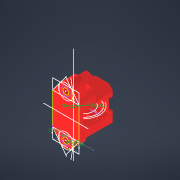
# Autodesk Inventor part: Front-Idlers_Inlet
Saved by Autodesk Inventor 2022.1 (Build 261234000, 234)
## iProperties
Created: 2021-09-01
Part Number: Front-Idlers_Inlet
Material: Generisch
Document SubType Name: Modeling
Designer: Rama
Density: 1 g/cm^3
Appearance: Hellrot
Author: Rama
Autodesk Inventor part; units mm, degrees
ref_plane "YZ Plane" through (0, 0, 0) normal (1, 0, 0) x (0, 1, 0)
ref_plane "XZ Plane" through (0, 0, 0) normal (0, 1, 0) x (-1, 0, 0)
ref_plane "XY Plane" through (0, 0, 0) normal (0, 0, 1) x (1, 0, 0)
sketch "Skizze1" plane through (0, 0, 0) normal (0, 0, 1) x (1, 0, 0)
  line L0 (-7.5, 9) -> (7.5, 9)
  line L1 (7.5, 9) -> (7.5, -9)
  line L2 (7.5, -9) -> (-7.5, -9)
  line L3 (-7.5, -9) -> (-7.5, 9)
  line L4 (-7.5, 9) -> (7.5, -9) construction
  line L5 (7.5, 9) -> (-7.5, -9) construction
  point P0 (0, 0)
  dimension "d0" = 15
  dimension "d1" = 18
  constraints: 12 end point, 2 midpoint, 2 parallel, 1 horizontal, 1 perpendicular
  measures "d0" distance of L1.end L2.end
  measures "d1" distance of L0.end L1.end
extrude "Extrusion1" add sketch "Skizze1" along normal blind 24
sketch "Skizze2" plane through (-7.5, 9, 0) normal (0, 1, 0) x (1, 0, 0)
  line L0 (0, -24) -> (15, -24) projected
  circle A0 centre (7.5, -14) radius 2.5
  point P0 (7.5, 0)
  dimension "d5" = 5
  dimension "d13" = 10
  constraints: 1 centre point
  measures "d5" diameter of A0
  measures "d13" distance from line of L0 A0.centre
extrude "Extrusion2" cut sketch "Skizze2" against normal through all
ref_plane "Arbeitsebene1" through (-7.5, 0, 0) normal (0, 1, 0) x (1, 0, 0)
sketch "Skizze3" plane through (-7.5, 0, 0) normal (0, 1, 0) x (1, 0, 0)
  circle A0 centre (7.5, -14) radius 2.5 projected
  circle A1 centre (7.5, -14) radius 8
  circle A2 centre (7.5, -14) radius 9
  line L0 (-1.5, -14) -> (16.5, -14)
  circle A3 centre (7.5, -14) radius 5
  line L1 (12.5, -14) -> (12.5, 0)
  line L2 (0, 0) -> (15, 0) projected
  line L3 (2.5, -14) -> (2.5, 0)
  line L4 (16.5, -14) -> (16.5, 0)
  line L5 (16.5, 0) -> (12.5, 0)
  line L6 (-1.5, -14) -> (-1.5, 0)
  line L7 (-1.5, 0) -> (2.5, 0)
  point P0 (7.5, 0)
  point P1 (15, 0)
  point P2 (12.5, -7.755)
  point P3 (2.5, -7.755)
  point P4 (0, 0)
  dimension "d8" = 16
  dimension "d9" = 18
  dimension "d10" = 10
  constraints: 14 end point, 5 point on line, 4 point on circle, 3 centre point, 3 coincident, 3 tangent, 2 parallel, 2 perpendicular, 1 collinear, 1 horizontal, 1 vertical
  measures "d8" diameter of A1
  measures "d9" diameter of A2
  measures "d10" diameter of A3
extrude "Extrusion3" cut sketch "Skizze3" against normal mid plane 10 contours L0 A3 A0 | A0 L0 A3 | L1 A1 L0 | L0 A1 A3 | A3 L3 A1 L1 | L0 A1 L3 | L0 A2 A1 | A1 L1 A2 L0 | L0 A2 L3 A1 | A2 L1 L2 L5 L4 | L6 L7 L2 L3 A2
sketch "Skizze4" plane through (-7.5, 9, 0) normal (0, 1, 0) x (1, 0, 0)
  line L0 (15, 0) -> (0, 0)
  line L1 (0, 0) -> (0, -4.5)
  line L2 (0, -4.5) -> (15, -4.5)
  line L3 (15, -4.5) -> (15, 0)
  circle A0 centre (7.5, -14) radius 2.5 projected
  line L4 (15, 0) -> (0, 0) projected
  line L5 (0, 0) -> (0, -24) projected
  line L6 (15, -24) -> (0, -24) projected
  line L7 (15, 0) -> (15, -24) projected
  line L8 (0, 0) -> (0, -24) projected
  line L9 (15, 0) -> (15, -24) projected
  line L10 (15, 0) -> (0, 0) projected
  line L11 (0, -18.9749) -> (0, 0) projected
  arc A1 (0, -18.9749) -> (15, -18.9749) centre (7.5, -14) ccw projected
  line L12 (15, 0) -> (15, -18.9749) projected
  line L13 (12.5, 0) -> (15, 0) projected
  line L14 (12.5, -7.755) -> (12.5, 0) projected
  arc A2 (12.5, -7.755) -> (2.5, -7.755) centre (7.5, -14) ccw projected
  line L15 (2.5, 0) -> (2.5, -7.755) projected
  line L16 (0, 0) -> (2.5, 0) projected
  circle A3 centre (7.5, -14) radius 2.5 projected
  point P0 (7.5, 0)
  point P1 (0, -2.25)
  point P2 (15, -2.25)
  point P3 (7.5, 0)
  dimension "d14" = 1.5
  constraints: 8 end point, 4 midpoint, 2 parallel, 2 point on line, 1 horizontal, 1 perpendicular
  measures "d14" distance edge to line of A2 L2
extrude "Extrusion4" cut sketch "Skizze4" against normal through all contours L3 L2 L14 L0 | L14 L2 L15 L0 | L15 L2 L1 L0
sketch "Skizze5" plane through (0, 0, 24) normal (0, 0, 1) x (1, 0, 0)
  line L0 (-3.5, 15) -> (3.5, 15)
  line L1 (3.5, 15) -> (3.5, -15)
  line L2 (3.5, -15) -> (-3.5, -15)
  line L3 (-3.5, -15) -> (-3.5, 15)
  line L4 (-3.5, 15) -> (3.5, -15) construction
  line L5 (3.5, 15) -> (-3.5, -15) construction
  line L6 (-7.5, -9) -> (7.5, -9) projected
  line L7 (7.5, -9) -> (7.5, 9) projected
  line L8 (7.5, 9) -> (-7.5, 9) projected
  line L9 (-7.5, 9) -> (-7.5, -9) projected
  point P0 (0, 0)
  point P1 (3.5, -9)
  point P2 (-3.5, -9)
  point P3 (-3.5, 9)
  point P4 (3.5, 9)
  dimension "d17" = 7
  dimension "d18" = 30
  constraints: 12 end point, 2 midpoint, 2 parallel, 1 horizontal, 1 perpendicular
  measures "d17" distance of L1.end L2.end
  measures "d18" distance of L0.end L1.end
extrude "Extrusion5" add sketch "Skizze5" against normal blind 7.5 contours L0 L1 L8 L3 | L6 L1 L2 L3
sketch "Skizze6" plane through (0, 0, 16.5) normal (0, 0, -1) x (-1, 0, 0)
  line L0 (3.5, 9) -> (3.5, 15) projected
  line L1 (3.5, 15) -> (-3.5, 15) projected
  line L2 (-3.5, 15) -> (-3.5, 9) projected
  line L3 (0, 9) -> (-3.5, 9) projected
  line L4 (3.5, 9) -> (0, 9) projected
  line L5 (-3.5, -9) -> (-3.5, -15) projected
  line L6 (-3.5, -15) -> (3.5, -15) projected
  line L7 (3.5, -15) -> (3.5, -9) projected
  line L8 (0, -9) -> (3.5, -9) projected
  line L9 (-3.5, -9) -> (0, -9) projected
  line L10 (3.5, 9) -> (3.5, 15) projected
  line L11 (-3.5, 9) -> (3.5, 9)
  line L12 (3.5, 9) -> (3.5, 15)
  line L13 (3.5, 15) -> (-3.5, 15)
  line L14 (-3.5, 15) -> (-3.5, 9)
  line L15 (-3.5, 9) -> (3.5, 15) construction
  line L16 (3.5, 9) -> (-3.5, 15) construction
  line L17 (-3.5, -15) -> (3.5, -15) projected
  line L18 (-3.5, -9) -> (3.5, -9)
  line L19 (3.5, -9) -> (3.5, -15)
  line L20 (3.5, -15) -> (-3.5, -15)
  line L21 (-3.5, -15) -> (-3.5, -9)
  line L22 (-3.5, -9) -> (3.5, -15) construction
  line L23 (3.5, -9) -> (-3.5, -15) construction
  point P0 (0, 0)
  point P1 (0, 12)
  point P2 (0, -12)
  constraints: 24 end point, 4 midpoint, 4 parallel, 2 horizontal, 2 perpendicular
hole "Bohrung1" at (0, 12, 16.5) at (0, -12, 16.5) direction (0, 0, 1) diameter 3.3 end through all counterbore diameter 4.8 counterbore depth 3.8
sketch "Skizze7" plane through (-7.5, 9, 4.5) normal (0, 1, 0) x (1, 0, 0)
  line L0 (5.6485, 8.9497) -> (5.6485, -0.1503)
  spline S0 degree 3 poles (5.6485, -0.1503) (5.6485, -0.2757) (5.6235, -0.4093) (5.5221, -0.6548) (5.4458, -0.7666) (5.2684, -0.9452) (5.1549, -1.0229) (4.9074, -1.1255) (4.7734, -1.1503) (4.6485, -1.1503) knots 0 0 0 0 0.247012 0.247012 0.494023 0.494023 0.747012 0.747012 1 1 1 1
  line L1 (2.6485, -1.1503) -> (4.6485, -1.1503)
  spline S1 degree 3 poles (2.4137, -1.1224) (2.359, -1.1092) (2.3053, -1.0913) (2.1283, -1.0152) (2.0153, -0.935) (1.845, -0.7571) (1.7725, -0.6496) (1.6741, -0.4099) (1.6485, -0.2772) (1.6485, -0.1503) knots 0 0 0 0 0.128043 0.128043 0.438246 0.438246 0.719123 0.719123 1 1 1 1
  spline S2 degree 3 poles (2.6485, -1.1503) (2.5718, -1.1503) (2.4922, -1.1413) (2.4137, -1.1224) knots 0 0 0 0 1 1 1 1
  line L2 (1.6485, -0.1503) -> (1.6485, 8.9497)
  spline S3 degree 3 poles (1.6485, 8.9497) (1.6485, 9.0766) (1.6741, 9.2092) (1.7725, 9.449) (1.845, 9.5564) (2.0153, 9.7344) (2.1283, 9.8145) (2.3053, 9.8906) (2.359, 9.9085) (2.4137, 9.9217) knots 0 0 0 0 0.280877 0.280877 0.561754 0.561754 0.871957 0.871957 1 1 1 1
  line L3 (4.6485, 9.9497) -> (2.6485, 9.9497)
  spline S4 degree 3 poles (4.6485, 9.9497) (4.7734, 9.9497) (4.9074, 9.9248) (5.1549, 9.8223) (5.2684, 9.7446) (5.4458, 9.566) (5.5221, 9.4541) (5.6235, 9.2086) (5.6485, 9.075) (5.6485, 8.9497) knots 0 0 0 0 0.252988 0.252988 0.505977 0.505977 0.752988 0.752988 1 1 1 1
  line L4 (5.6485, 8.9497) -> (5.6485, -0.1503)
  spline S5 degree 3 poles (2.4137, 9.9217) (2.4922, 9.9407) (2.5718, 9.9497) (2.6485, 9.9497) knots 0 0 0 0 1 1 1 1
  point P0 (7.5, 4.5)
extrude "Extrusion6" cut sketch "Skizze7" against normal through all
chamfer "Fase1" distance 1 angle 45 8 edges at (2.8243, -9, 4.5) (2.8243, 9, 4.5) (-6.6757, -9, 4.5) (-6.6757, 9, 4.5) (7.5, 7, 4.5) (7.5, -7, 4.5) (-7.5, -7, 4.5) (-7.5, 7, 4.5)
move faces "Verschieben1" translate (0, -0.05, 0) faces at (-4.9758, -5, 13.3772)
move faces "Verschieben2" translate (0, 0.05, 0) faces at (-4.9758, 5, 13.3772)
sketch "Skizze8" plane through (6.5, 8, 4.5) normal (0, 0, -1) x (-1, 0, 0)
  line L0 (0, 0) -> (8.3515, 0) projected
  line L1 (0, -2.95) -> (0, 0) projected
  line L2 (1.5, -2.95) -> (0, -2.95) projected
  line L3 (1.5, -13.05) -> (1.5, -2.95) projected
  line L4 (0, -13.05) -> (1.5, -13.05) projected
  line L5 (0, -16) -> (0, -13.05) projected
  line L6 (8.3515, -16) -> (0, -16) projected
  line L7 (8.3515, -16) -> (8.3515, 0) projected
  line L8 (-1, 1) -> (-1, -2.95) projected
  line L9 (-1, -2.95) -> (0, -2.95) projected
  line L10 (0, -2.95) -> (0, 0) projected
  line L11 (0, 0) -> (-1, 1) projected
  line L12 (0, 0) -> (8.3515, 0) projected
  line L13 (8.3515, 0) -> (8.3515, 0.1503) projected
  line L14 (8.8247, 1) -> (-1, 1) projected
  line L15 (0, 0) -> (-1, 1) projected
  line L16 (0, 0) -> (-1, 1) projected
  line L17 (-1, 1) -> (2, 1)
  line L18 (2, 1) -> (2, -2)
  line L19 (2, -2) -> (-1, -2)
  line L20 (-1, -2) -> (-1, 1)
  line L21 (-1, -2) -> (2, 1)
  point P0 (6.5, -8)
  point P1 (-1, -2)
  dimension "d46" = 3
  dimension "d47" = 3
  constraints: 10 end point, 2 parallel, 1 horizontal, 1 perpendicular, 1 other
  measures "d46" distance of L18.end L19.end
  measures "d47" distance of L17.end L18.end
extrude "Extrusion7" cut sketch "Skizze8" against normal blind 10 contours L11 L14 L21 L0 | L0 L21 L1 | L1 L21 L8 L11
delete faces "Fläche löschen1" heal yes whole lump no faces at (7.1667, -7.35, 5.1667) (6.8333, 6.0167, 4.8333) (-7.1667, -7.35, 5.1667) (-7.1667, 7.35, 5.1667)
delete faces "Fläche löschen2" heal yes whole lump no faces at (4.3769, -8.4456, 4.9456) (-6.9348, -8.4843, 4.9843) (2.7162, 8.3333, 4.8333) (-6.9348, 8.4843, 4.9843)
chamfer "Fase8" distance 0.4 angle 45 6 edges at (-6.6757, -9, 4.5) (-6.6757, 9, 4.5) (7.5, -6.525, 4.5) (7.5, -8.5, 4.5) (7.5, 5.525, 4.5) (1.3243, 9, 4.5)
move faces "Verschieben9" translate (0, 0.25, 0) faces at (-6.401, 5.05, 15.1545) (-6.9505, 5.05, 4.9335) (4.976, 5.05, 13.3782) (-5.6566, 5.05, 5.4487) (-2.057, 5.05, 6.3328) (-5.0288, 5.05, 5.6349)
move faces "Verschieben10" translate (0, -0.25, 0) faces at (-6.401, -5.05, 15.1545) (-6.9505, -5.05, 4.9335) (-4.4505, -5.05, 14.1977) (-5.6566, -5.05, 5.4487) (-2.057, -5.05, 6.3328) (-5.0288, -5.05, 5.6349)
sketch "Skizze11" plane through (0, 0, 24) normal (0, 0, 1) x (1, 0, 0)
  circle A0 centre (0, 12) radius 1.65 projected
  line L0 (-7.5, 9) -> (-7.5, -9) projected
  line L1 (-7.5, -9) -> (-3.5, -9) projected
  line L2 (-3.5, -9) -> (-3.5, -15) projected
  line L3 (-3.5, -15) -> (3.5, -15) projected
  line L4 (3.5, -15) -> (3.5, -9) projected
  line L5 (3.5, -9) -> (7.5, -9) projected
  line L6 (7.5, -9) -> (7.5, 9) projected
  line L7 (7.5, 9) -> (3.5, 9) projected
  line L8 (3.5, 9) -> (3.5, 15) projected
  line L9 (3.5, 15) -> (-3.5, 15) projected
  line L10 (-3.5, 15) -> (-3.5, 9) projected
  line L11 (-3.5, 9) -> (-7.5, 9) projected
  circle A1 centre (0, -12) radius 1.65 projected
  circle A2 centre (0, -12) radius 2.4
  circle A3 centre (0, -12) radius 1.65 projected
  circle A4 centre (0, -12) radius 4.2
  line L12 (7.5, -9) -> (7.5, 9) projected
  line L13 (7.5, -9) -> (-1.8834, -9) projected
  line L14 (7.5, -9) -> (-0.1662, -19.2215)
  line L15 (-7.5, -9) -> (-7.5, -5.3) projected
  line L16 (-7.1, -8.6) -> (-7.5, -9) projected
  line L17 (-7.5, -9) -> (0.4202, -19.5603)
  line L18 (7.5, -15) -> (-7.5, -15)
  line L19 (-7.5, -15) -> (-7.5, -9)
  line L20 (-7.5, -9) -> (7.5, -9)
  line L21 (7.5, -9) -> (7.5, -15)
  line L22 (7.5, -15) -> (-7.5, -9) construction
  line L23 (-7.5, -15) -> (7.5, -9) construction
  line L24 (12.4621, 0) -> (-12.5573, 0)
  circle A5 centre (0, 12) radius 2.4
  circle A6 centre (0, 12) radius 4.2
  line L25 (7.5, 9) -> (-0.1662, 19.2215)
  line L26 (-7.5, 9) -> (0.4202, 19.5603)
  line L27 (7.5, 15) -> (-7.5, 15)
  line L28 (-7.5, 15) -> (-7.5, 9)
  line L29 (-7.5, 9) -> (7.5, 9)
  line L30 (7.5, 9) -> (7.5, 15)
  line L31 (4.2, -19.7874) -> (4.2, 35)
  line L32 (-7.5, 9) -> (-7.5, -9) projected
  line L33 (3.5, -9) -> (7.5, -9) projected
  line L34 (4.7938, -9) -> (2.8475, -20.0377)
  line L35 (4.7938, -9) -> (16.0017, -9) construction
  line L36 (4.7938, 9) -> (2.8475, 20.0377)
  point P0 (0, 0)
  point P1 (-7.5, -8.6)
  point P2 (-2.9394, 15)
  point P3 (2.9394, 15)
  point P4 (2.9394, -15)
  point P5 (-2.9394, -15)
  point P6 (-3.5, 14.3216)
  point P7 (-3.36, 14.52)
  point P8 (-3.36, -14.52)
  point P9 (-3.5, -14.3216)
  point P10 (3.5, -14.3216)
  point P11 (4.4, -12)
  point P12 (4.2, -9)
  point P13 (4.2, 12)
  point P14 (3.5, 14.3216)
  point P15 (4.2, 9)
  point P16 (7.5, -12)
  point P17 (-7.5, -12)
  point P18 (0, -9)
  point P19 (4.2, -12)
  point P20 (3.5, -9.6784)
  point P21 (-3.5, 9.6784)
  point P22 (3.5, 9.6784)
  point P23 (-3.5, -9.6784)
  point P24 (-3.36, -14.52)
  point P25 (-3.36, 14.52)
  point P26 (2.9394, 9)
  point P27 (-2.9394, 9)
  point P28 (-2.9394, -9)
  point P29 (2.9394, -9)
  point P30 (4.2, -13.4)
  point P31 (3.5, -14.3333)
  point P32 (-3.5, 14.3333)
  point P33 (-3, 15)
  point P34 (4.2, 12.3675)
  point P35 (4.2, -12.3675)
  point P36 (3.5, 14.3333)
  point P37 (3.36, 14.52)
  point P38 (4.1362, 12.7293)
  point P39 (4.1362, -12.7293)
  dimension "d106" = 8.4
  dimension "d107" = 53.13
  dimension "d109" = 53.13
  dimension "d123" = 100
  constraints: 38 end point, 11 symmetric about line, 5 midpoint, 5 point on line, 3 centre point, 3 horizontal, 3 parallel, 2 coincident, 2 vertical, 1 equal length, 1 perpendicular, 8 other
  measures "d107" angle of L5 L14
  measures "d109" angle of L17 L1
  measures "d123" angle of L34 L35
extrude "Extrusion9" add sketch "Skizze11" against normal up to surface (7.5 mm away) contours L1 L2 A4 L17 | L20 A4 L2 | L2 A4 L17 | L26 L10 A6 L11 | A4 L20 L13 L4 L3 L2 | L2 A4 | A4 L13 L20 | L10 A6 L29 | L26 A6 L10 | L31 A4 L4 L5 | L5 L34 L31 | L31 L36 L7 | L7 L8 A6 L31 | L13 L4 A4 | L3 A4 | A6 L10 | L10 A6 L9 L8 L29 | L29 A6 | A4 L4 | L31 L34 A4 | L29 A6 L8 | A6 L8 | A6 L36 L31 | A6 L9
extrude "Extrusion10" cut sketch "Skizze11" against normal through all contours L17 L3 L2 | L2 A4 L17 | A4 L3 L17 | L26 A6 L10 | L10 L9 L26 | L26 L9 A6 | A4 L14 L3 | L14 L34 L31 | L34 L14 L4 A4 | L4 L14 A4 | L14 L4 L3 | L9 L25 A6 | A6 L25 L8 | L9 L8 L25
chamfer "Fase10" distance 0.4 angle 45 1 edges at (-7.5, 0, 24)
sketch "Skizze13" plane through (7.1, -9, 4.5) normal (0, 0, -1) x (-1, 0, 0)
  line L0 (0, 3.7) -> (2.1, 3.7) projected
  line L1 (0, 0) -> (0, 3.7) projected
  line L2 (8.9515, 0) -> (0, 0) projected
  line L3 (8.9515, 0) -> (8.9515, 17.6) projected
  line L4 (2.2, 17.6) -> (8.9515, 17.6) projected
  line L5 (2.2, 17.6) -> (0, 15.4) projected
  line L6 (0, 14.3) -> (0, 15.4) projected
  line L7 (2.1, 14.3) -> (0, 14.3) projected
  line L8 (2.1, 3.7) -> (2.1, 14.3) projected
  line L9 (4, 0) -> (3.1071, 0.8929)
  line L10 (4, 0) -> (5.2627, 0) construction
  line L11 (1.6929, 0.8929) -> (0.8, 0)
  line L12 (0.8, 0) -> (4, 0)
  line L13 (8.9515, 0) -> (0, 0) projected
  arc A0 (3.1071, 0.8929) -> (1.6929, 0.8929) centre (2.4, 0.1858) ccw
  point P0 (7.1, 9)
  point P1 (2.4, 1.6)
  point P2 (2.4, 0)
  point P3 (0.8, 0)
  point P4 (4, 0)
  dimension "d124" = 135
  dimension "d125" = 90
  dimension "d126" = 1.6
  dimension "d127" = 0.8
  dimension "d128" = 1
  constraints: 8 end point, 3 point on line, 2 horizontal, 2 point on circle, 2 tangent, 1 centre point, 1 equal length, 1 midpoint
  measures "d124" angle of L10 L9
  measures "d125" angle of L11 L9
  measures "d126" distance from line of L2 point (2.4, 1.6)
  measures "d127" distance from line of L11.end L1
  measures "d128" radius of A0
extrude "Extrusion13" cut sketch "Skizze13" against normal blind 10.5 contours L11 A0 L9 L2
sketch "Skizze18" plane through (0, -5.3, 14) normal (0, 1, 0) x (1, 0, 0)
  line L0 (7.1, 9.5) -> (7.5, 9.1) projected
  line L1 (7.1, 9.5) -> (5, 9.5) projected
  line L2 (5, 6.245) -> (5, 9.5) projected
  arc A0 (5, 6.245) -> (-5, 6.245) centre (0, 0) ccw projected
  line L3 (-5, 8.3608) -> (-5, 6.245) projected
  arc A1 (-5.0863, 8.3776) -> (-5, 8.3608) centre (-4.8509, 9.3547) ccw projected
  spline S0 degree 5 poles (-5.0863, 8.3776) (-5.0877, 8.378) (-5.0887, 8.3782) (-5.0895, 8.3784) (-5.0902, 8.3786) (-5.1064, 8.3826) (-5.1218, 8.3867) (-5.1372, 8.3912) (-5.1524, 8.3959) (-5.1841, 8.4065) (-5.2006, 8.4124) (-5.217, 8.4186) (-5.2332, 8.4252) (-5.2868, 8.4485) (-5.3234, 8.4667) (-5.3591, 8.4869) (-5.3937, 8.5087) (-5.4875, 8.5748) (-5.5441, 8.6226) (-5.5959, 8.6757) (-5.6422, 8.7335) (-5.7484, 8.8927) (-5.8, 8.9998) (-5.8337, 9.1146) (-5.851, 9.2321) (-5.8515, 9.3497) knots 0 0 0 0 0 0 0.002968 0.002968 0.002968 0.002968 0.062827 0.062827 0.062827 0.062827 0.128504 0.128504 0.128504 0.128504 0.281952 0.281952 0.281952 0.281952 0.558819 0.558819 0.558819 0.558819 1 1 1 1 1 1 projected
  line L4 (-5.8515, 9.3497) -> (-5.8515, 9.5) projected
  line L5 (-5.8515, 9.5) -> (-7.5, 9.5) projected
  line L6 (-7.5, -4.9749) -> (-7.5, 9.5) projected
  arc A2 (-7.5, -4.9749) -> (7.5, -4.9749) centre (0, 0) ccw projected
  line L7 (7.5, 9.1) -> (7.5, -4.9749) projected
  circle A3 centre (0, 0) radius 2.5 projected
  point P0 (0, 14)
  constraints: 1 other
extrude "Extrusion19" add sketch "Skizze18" along normal blind 3
sketch "Skizze19" plane through (0, 5.3, 14) normal (0, -1, 0) x (1, 0, 0)
  line L0 (7.5, -9.1) -> (7.1, -9.5) projected
  line L1 (7.5, 4.9749) -> (7.5, -9.1) projected
  arc A0 (7.5, 4.9749) -> (-7.5, 4.9749) centre (0, 0) ccw projected
  line L2 (-7.5, -9.5) -> (-7.5, 4.9749) projected
  line L3 (-7.5, -9.5) -> (-5.8515, -9.5) projected
  line L4 (-5.8515, -9.5) -> (-5.8515, -9.3497) projected
  spline S0 degree 5 poles (-5.8515, -9.3497) (-5.851, -9.2321) (-5.8337, -9.1146) (-5.8, -8.9998) (-5.7484, -8.8927) (-5.6422, -8.7335) (-5.5959, -8.6757) (-5.5441, -8.6226) (-5.4875, -8.5748) (-5.3937, -8.5087) (-5.3591, -8.4869) (-5.3234, -8.4667) (-5.2868, -8.4485) (-5.2332, -8.4252) (-5.217, -8.4186) (-5.2006, -8.4124) (-5.1841, -8.4065) (-5.1524, -8.3959) (-5.1372, -8.3912) (-5.1218, -8.3867) (-5.1064, -8.3826) (-5.0902, -8.3786) (-5.0895, -8.3784) (-5.0887, -8.3782) (-5.0877, -8.378) (-5.0863, -8.3776) knots 0 0 0 0 0 0 0.441181 0.441181 0.441181 0.441181 0.718048 0.718048 0.718048 0.718048 0.871496 0.871496 0.871496 0.871496 0.937173 0.937173 0.937173 0.937173 0.997032 0.997032 0.997032 0.997032 1 1 1 1 1 1 projected
  arc A1 (-5, -8.3608) -> (-5.0863, -8.3776) centre (-4.8509, -9.3547) ccw projected
  line L5 (-5, -6.245) -> (-5, -8.3608) projected
  arc A2 (-5, -6.245) -> (5, -6.245) centre (0, 0) ccw projected
  line L6 (5, -9.5) -> (5, -6.245) projected
  line L7 (5, -9.5) -> (7.1, -9.5) projected
  circle A3 centre (0, 0) radius 2.5 projected
  point P0 (0, -14)
  constraints: 1 other
extrude "Extrusion20" add sketch "Skizze19" along normal blind 3
sketch "Skizze20" plane through (-7.5, 0, 0) normal (0, 1, 0) x (1, 0, 0)
  circle A0 centre (7.5, -14) radius 2.08
  circle A1 centre (7.5, -14) radius 5.5
  circle A2 centre (7.5, -14) radius 8
  circle A3 centre (7.5, -14) radius 9
  line L0 (-1.5, -14) -> (16.5, -14)
  point P0 (7.5, 0)
  point P1 (13, -14)
  point P2 (2, -14)
  dimension "d188" = 11
  dimension "d189" = 16
  dimension "d190" = 18
  constraints: 4 centre point, 3 coincident, 2 end point, 2 point on circle, 1 horizontal, 2 other
  measures "d188" diameter of A1
  measures "d189" diameter of A2
  measures "d190" diameter of A3
extrude "Extrusion21" cut sketch "Skizze20" along normal mid plane 10.5 contours L0 A0 | L0 A1 A0 | A0 L0 A1 | A0 L0
extrude "Extrusion22" cut sketch "Skizze20" along normal mid plane 9.5 contours L0 A0 | L0 A1 A0 | A0 L0 A1 | A0 L0 | L0 A2 A1 | A1 L0 A2
extrude "Extrusion23" cut sketch "Skizze20" along normal mid plane 7.2 contours L0 A2 A1 | L0 A3 A2 picked at (14.5892, -14.6382) picked at (16.0795, -14.7179)
sketch "Skizze21" plane through (-7.5, 0, 0) normal (0, 1, 0) x (1, 0, 0)
  arc A0 (15, -11.2161) -> (12.5, -7.755) centre (7.5, -14) ccw projected
  line L0 (15, -11.2161) -> (15, -4.9) projected
  line L1 (15, -4.9) -> (14.6, -4.5) projected
  line L2 (14.6, -4.5) -> (12.5, -4.5) projected
  line L3 (12.5, -7.755) -> (12.5, -4.5) projected
  arc A1 (2.5, -7.755) -> (0, -11.2161) centre (7.5, -14) ccw projected
  line L4 (2.5, -5.6392) -> (2.5, -7.755) projected
  arc A2 (2.4137, -5.6224) -> (2.5, -5.6392) centre (2.6491, -4.6453) ccw projected
  spline S0 degree 5 poles (2.4137, -5.6224) (2.4123, -5.622) (2.4113, -5.6218) (2.4105, -5.6216) (2.4098, -5.6214) (2.3936, -5.6174) (2.3782, -5.6133) (2.3628, -5.6088) (2.3476, -5.6041) (2.3159, -5.5935) (2.2994, -5.5876) (2.283, -5.5814) (2.2668, -5.5748) (2.2132, -5.5515) (2.1766, -5.5333) (2.1409, -5.5131) (2.1063, -5.4913) (2.0125, -5.4252) (1.9559, -5.3774) (1.9041, -5.3243) (1.8578, -5.2665) (1.7516, -5.1073) (1.7, -5.0002) (1.6663, -4.8854) (1.649, -4.7679) (1.6485, -4.6503) knots 0 0 0 0 0 0 0.002968 0.002968 0.002968 0.002968 0.062827 0.062827 0.062827 0.062827 0.128504 0.128504 0.128504 0.128504 0.281952 0.281952 0.281952 0.281952 0.558819 0.558819 0.558819 0.558819 1 1 1 1 1 1 projected
  line L5 (1.6485, -4.6503) -> (1.6485, -4.5) projected
  line L6 (1.6485, -4.5) -> (0, -4.5) projected
  line L7 (0, -4.5) -> (0, -11.2161) projected
  point P0 (7.5, 0)
  constraints: 1 other
extrude "Extrusion24" cut sketch "Skizze21" along normal mid plane 7.2
sketch "Skizze22" plane through (7.5, -9, 24) normal (1, 0, 0) x (0, 0, -1)
  line L0 (12.5, 3.75) -> (7.5, 3.75) projected
  line L1 (12.5, 0) -> (7.5, 0) projected
  line L2 (19.1, 0) -> (0, 0) projected
  line L3 (9.5, 18) -> (0, 18) projected
  line L4 (2.5, 13) -> (17.5, 13)
  line L5 (17.5, 13) -> (17.5, 5)
  line L6 (17.5, 5) -> (2.5, 5)
  line L7 (2.5, 5) -> (2.5, 13)
  line L8 (2.5, 13) -> (17.5, 5) construction
  line L9 (17.5, 13) -> (2.5, 5) construction
  point P0 (24, 9)
  point P1 (10, 9)
  dimension "d199" = 5
  dimension "d200" = 18
  dimension "d201" = 9
  dimension "d203" = 2.5
  dimension "d204" = 8
  dimension "d205" = 15
  constraints: 12 end point, 2 midpoint, 2 parallel, 1 horizontal, 1 perpendicular
  measures "d199" distance of L0.start L0.end
  measures "d200" distance between parallel lines of L2 L3
  measures "d201" distance from line of L3 point (10, 9)
  measures "d203" horizontal distance of L0.end point (10, 9)
  measures "d204" distance of L4.end L5.end
  measures "d205" distance of L4.start L4.end
extrude "Extrusion25" cut sketch "Skizze22" against normal blind 7.5
chamfer "Fase22" distance 0.4 angle 45 4 edges at (6.25, -3.6, 6.5) (6.25, 3.6, 6.5) (3.8794, -3.6, 21.5) (3.8794, 3.6, 21.5)
chamfer "Fase23" distance 0.5 angle 45 2 edges at (-5.5, -4.75, 14) (-5.5, 4.75, 14)
fillet "Rundung12" radius 4 5 edges at (4.9749, -3.7999, 21.5) (4.9749, -2.95, 21.5) (4.9749, 0, 21.5) (4.9749, 2.95, 21.5) (4.9749, 3.8, 21.5)
fillet "Rundung13" radius 4 4 edges at (2.7839, 3.15, 6.5) (2.7839, -3.15, 6.5) (2.7839, -1.15, 6.5) (2.7839, 1.15, 6.5)
sketch "Skizze23" plane through (-7.5, 0, 0) normal (0, 1, 0) x (1, 0, 0)
  arc A0 (15, -11.2161) -> (9.7852, -6.3333) centre (7.5, -14) ccw projected
  line L0 (15, -6.5) -> (15, -11.2161) projected
  line L1 (15, -6.5) -> (12.5, -6.5) projected
  line L2 (12.5, -6.5) -> (10.9278, -6.5) projected
  arc A1 (9.7852, -6.3333) -> (10.9278, -6.5) centre (10.9278, -2.5) ccw projected
  arc A2 (10.2839, -21.5) -> (15, -16.7839) centre (7.5, -14) ccw projected
  line L3 (13.5622, -21.5) -> (10.2839, -21.5) projected
  line L4 (15, -21.5) -> (13.5622, -21.5) projected
  line L5 (15, -16.7839) -> (15, -21.5) projected
  line L6 (15, -11.2161) -> (15, -16.7839) projected
  line L7 (15, -16.7839) -> (14.2, -16.7839)
  line L8 (14.2, -16.7839) -> (14.2, -17.5839)
  line L9 (14.2, -17.5839) -> (15, -17.5839)
  line L10 (15, -17.5839) -> (15, -16.7839)
  line L11 (15, -6.5) -> (15, -11.2161) projected
  line L12 (15, -11.2161) -> (14.2, -11.2161)
  line L13 (14.2, -11.2161) -> (14.2, -10.4161)
  line L14 (14.2, -10.4161) -> (15, -10.4161)
  line L15 (15, -10.4161) -> (15, -11.2161)
  point P0 (7.5, 0)
  point P1 (14.6523, -10.4161)
  point P2 (14.6523, -17.5839)
  dimension "d216" = 0.8
  dimension "d217" = 0.8
  dimension "d218" = 0.8
  dimension "d219" = 0.8
  constraints: 16 end point, 4 parallel, 2 horizontal, 2 perpendicular
  measures "d216" distance of L9.end L8.end
  measures "d217" distance of L8.end L7.end
  measures "d218" distance of L13.end L14.end
  measures "d219" distance of L12.end L13.end
extrude "Extrusion26" cut sketch "Skizze23" against normal mid plane 9.5 contours A0 L14 L0 | A2 L5 L9
chamfer "Fase24" distance 0.4 angle 45 3 edges at (5, 3.15, 6.5) (5, 0, 6.5) (5, -3.1499, 6.5)
sketch "Skizze24" plane through (-7.5, 0, 0) normal (0, 1, 0) x (1, 0, 0)
  line L0 (1.6485, -4.5) -> (1.6485, -4.6503) projected
  line L1 (0, -4.5) -> (1.6485, -4.5) projected
  line L2 (0, -11.2161) -> (0, -4.5) projected
  arc A0 (2.5, -7.755) -> (0, -11.2161) centre (7.5, -14) ccw projected
  line L3 (2.5, -5.6392) -> (2.5, -7.755) projected
  arc A1 (2.4137, -5.6224) -> (2.5, -5.6392) centre (2.6491, -4.6453) ccw projected
  line L4 (8.761, -21.9) -> (11.8186, -21.9) projected
  arc A2 (0, -16.7839) -> (8.761, -21.9) centre (7.5, -14) ccw projected
  line L5 (0, -18.9749) -> (0, -16.7839) projected
  arc A3 (0, -18.9749) -> (11.6969, -21.9615) centre (7.5, -14) ccw projected
  arc A4 (11.8186, -21.9) -> (11.6969, -21.9615) centre (13.5622, -25.5) ccw projected
  arc A5 (2.5, -7.755) -> (0, -11.2161) centre (7.5, -14) ccw projected
  line L6 (0, -11.2161) -> (0.8, -11.2161)
  line L7 (0.8, -11.2161) -> (0.8, -10.4161)
  line L8 (0.8, -10.4161) -> (0, -10.4161)
  line L9 (0, -10.4161) -> (0, -11.2161)
  line L10 (0, -18.9749) -> (0, -16.7839) projected
  line L11 (0, -16.7839) -> (0.8, -16.7839)
  line L12 (0.8, -16.7839) -> (0.8, -17.5839)
  line L13 (0.8, -17.5839) -> (0, -17.5839)
  line L14 (0, -17.5839) -> (0, -16.7839)
  point P0 (7.5, 0)
  point P1 (0.3477, -17.5839)
  point P2 (0.3477, -10.4161)
  point P3 (0, -10.4161)
  dimension "d225" = 0.8
  dimension "d226" = 0.8
  dimension "d227" = 0.8
  dimension "d228" = 0.8
  constraints: 16 end point, 4 parallel, 2 horizontal, 2 perpendicular, 1 other
  measures "d225" distance of L8.end L7.end
  measures "d226" distance of L7.end L6.end
  measures "d227" distance of L12.end L13.end
  measures "d228" distance of L11.end L12.end
extrude "Extrusion27" cut sketch "Skizze24" against normal mid plane 9.5 contours L2 L8 A0 | L13 L5 A2
sketch "Skizze25" plane through (-7.5, -3.6, 0) normal (0, 1, 0) x (1, 0, 0)
  line L0 (0.3477, -17.5839) -> (0, -17.5839) projected
  line L1 (0, -18.9749) -> (0, -17.5839) projected
  arc A0 (0, -18.9749) -> (11.6969, -21.9615) centre (7.5, -14) ccw projected
  arc A1 (11.8186, -21.9) -> (11.6969, -21.9615) centre (13.5622, -25.5) ccw projected
  line L2 (8.761, -21.9) -> (11.8186, -21.9) projected
  arc A2 (0.3477, -17.5839) -> (8.761, -21.9) centre (7.5, -14) ccw projected
  line L3 (0, -18.9749) -> (0, -17.5839) projected
  line L4 (0, -18.9749) -> (0.8, -18.9749)
  line L5 (0.8, -18.9749) -> (0.8, -19.7749)
  line L6 (0.8, -19.7749) -> (0, -19.7749)
  line L7 (0, -19.7749) -> (0, -18.9749)
  point P0 (7.5, 0)
  point P1 (0.5971, -19.7749)
  dimension "d231" = 0.8
  dimension "d232" = 0.8
  constraints: 8 end point, 2 parallel, 1 horizontal, 1 perpendicular
  measures "d231" distance of L5.end L6.end
  measures "d232" distance of L4.end L5.end
extrude "Extrusion28" cut sketch "Skizze25" along normal up to surface (7.2 mm away) contours A0 L6 L7
chamfer "Fase25" distance 0.4 angle 45 2 edges at (-3.6513, -3.6, 21.1181) (-3.6513, 3.6, 21.1181)
fillet "Rundung14" radius 0.4 4 edges at (-5, -2.95, 7.755) (-5, 2.95, 7.755) (-5, 1.15, 7.755) (-5, -1.15, 7.755)
sketch "Skizze26" plane through (-7.5, 0, 0) normal (0, 1, 0) x (1, 0, 0)
  circle A0 centre (7.5, -14) radius 2.5 projected
  circle A1 centre (7.5, -14) radius 2.575
  point P0 (7.5, 0)
  point P1 (7.5, -16.5)
  dimension "d239" = 5.15
  constraints: 1 centre point, 1 coincident, 1 vertical alignment
  measures "d239" diameter of A1
extrude "Extrusion29" cut sketch "Skizze26" along normal mid plane 18 contours A0 | A1
delete faces "Fläche löschen5" heal yes whole lump no faces at (0.0691, 9, 16.5222)
delete faces "Fläche löschen6" heal yes whole lump no faces at (0.0691, -9, 16.5222)
